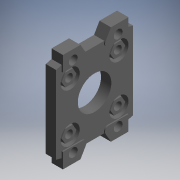
# Autodesk Inventor part: CA1-F06(F)
Saved by Autodesk Inventor 2017.3 (Build 213256000, 256)
## iProperties
Part Number: CA1-F06(F)
Material: Generic
Catalog Web Link: www.cadenas.de
Description: CE2 FLANGE-Stroke Reading Cylinder with Brake
Vendor: SMC
Document SubType Name: Modeling
Designer: partserver
Manufacturer: SMC
Mass: 122.984 g
Surface Area: 369.351 cm^2
Volume: 122.984 cm^3
Density: 1 g/cm^3
Appearance: PSOLRGB-128-128-128
Category: PARTsolutions
Company: SMC
Title: CA1-F06
Author: Cadenas PARTsolutions
Comments: Stroke Reading Cylinder with Brake
PSOL_IDENT_0: {$CADENAS_DATA\23d-libs\smc_jp\actuator\stroke_reading_cylinders\ce2\parts\ce2_flange.prj},166 {VTYP=
PSOL_IDENT_1: 3D},{NB=CA1-F06(F)},{LINA=CA1-F06},{NN=CE2 FLANGE},{DATE=05.07.2021 01:49:17},{GEOMDATE=15.05.2019 0
PSOL_IDENT_2: 8:14:22},{VERSION=},{LINEID=80},{WBVAR=MOUNT},{WBNUMERIC=}  {NB=CA1-F06(F)},{LINA=CA1-F06},{KT=DUMMY
PSOL_IDENT_3: },{PARTNO=CA1-F06},{BORE=63},{MOUNT=F},{B=85},{C=64},{D=20},{E=40},{J=M10x1.25},{JN=10},{FB=101},{FV=
PSOL_IDENT_4: 86},{FD=11.5},{FT=15},{FX=105},{FY=59},{FZ=130},{NM=6.0},{NS=17},{WM=2.0},{WD=8.70},{FT2=13.5},{FT3=
PSOL_IDENT_5: 4},{FB2=40},{FR=5},{FX2=90.2},{FZ2=102.0},{FA=75},{D0=44.000}
NB: CA1-F06(F)
NN: CE2 FLANGE
NT: Stroke Reading Cylinder with Brake
NBSYN: $PARTNO.($MOUNT.)
LINA: CA1-F06
CATALOG: SMC (JP
PARTNO: CA1-F06
BORE: 63
MOUNT: (F) Rod side flange style
B: 85
C: 64
D: 20
E: 40
J: M10x1.25
JN: 10
FB: 101
FV: 86
FD: 11.5
FT: 15
FX: 105
FY: 59
FZ: 130
NM: 6
NS: 17
WM: 2
WD: 8.7
FT2: 13.5
FT3: 4
FB2: 40
FR: 5
FX2: 90.2
FZ2: 102
FA: 75
D0: 44
SUPPLIER: SMC
ARTICLENO: CA1-F06(F)
BOMINFO: CA1-F06
CREATOR: CADENAS GmbH
Autodesk Inventor part; units mm, degrees
sketch "Sketch_1" plane through (0, 0, 0) normal (1, 0, 0) x (0, 1, 0)
  line L0 (43, 53.0096) -> (43, 52.5)
  line L1 (43, 52.5) -> (-43, 52.5)
  line L2 (-43, 52.5) -> (-43, 53.0096)
  line L3 (-43, 53.0096) -> (-50.5, 51)
  line L4 (-50.5, 51) -> (-50.5, -51)
  line L5 (-50.5, -51) -> (-43, -53.0096)
  line L6 (-43, -53.0096) -> (-43, -52.5)
  line L7 (-43, -52.5) -> (43, -52.5)
  line L8 (43, -52.5) -> (43, -53.0096)
  line L9 (43, -53.0096) -> (50.5, -51)
  line L10 (50.5, -51) -> (50.5, 51)
  line L11 (50.5, 51) -> (43, 53.0096)
  circle A0 centre (0, 0) radius 22
  constraints: 24 end point, 1 centre point
extrude "Extrusion1" add sketch "Sketch_1" against normal blind 13.5
sketch "Sketch_2" plane through (0, 0, 0) normal (1, 0, 0) x (0, 1, 0)
  line L0 (-17.171, -45.1) -> (-43, -45.1)
  line L1 (-43, -45.1) -> (-43, -65)
  line L2 (-43, -65) -> (-20, -65)
  line L3 (-20, -65) -> (-12.8409, -52.6)
  arc A0 (-12.8409, -52.6) -> (-17.171, -45.1) centre (-17.171, -50.1) ccw
  constraints: 8 end point, 2 point on circle, 1 centre point
extrude "Extrusion2" add sketch "Sketch_2" against normal blind 15
sketch "Sketch_3" plane through (0, 0, 0) normal (1, 0, 0) x (0, 1, 0)
  arc A0 (17.171, -45.1) -> (12.8409, -52.6) centre (17.171, -50.1) ccw
  line L0 (12.8409, -52.6) -> (20, -65)
  line L1 (20, -65) -> (43, -65)
  line L2 (43, -65) -> (43, -45.1)
  line L3 (43, -45.1) -> (17.171, -45.1)
  constraints: 8 end point, 2 point on circle, 1 centre point
extrude "Extrusion3" add sketch "Sketch_3" against normal blind 15
sketch "Sketch_4" plane through (0, 0, 0) normal (1, 0, 0) x (0, 1, 0)
  line L0 (-20, 65) -> (-43, 65)
  line L1 (-43, 65) -> (-43, 45.1)
  line L2 (-43, 45.1) -> (-17.171, 45.1)
  arc A0 (-17.171, 45.1) -> (-12.8409, 52.6) centre (-17.171, 50.1) ccw
  line L3 (-12.8409, 52.6) -> (-20, 65)
  constraints: 8 end point, 2 point on circle, 1 centre point
extrude "Extrusion4" add sketch "Sketch_4" against normal blind 15
sketch "Sketch_5" plane through (0, 0, 0) normal (1, 0, 0) x (0, 1, 0)
  line L0 (20, 65) -> (12.8409, 52.6)
  arc A0 (12.8409, 52.6) -> (17.171, 45.1) centre (17.171, 50.1) ccw
  line L1 (17.171, 45.1) -> (43, 45.1)
  line L2 (43, 45.1) -> (43, 65)
  line L3 (43, 65) -> (20, 65)
  constraints: 8 end point, 2 point on circle, 1 centre point
extrude "Extrusion5" add sketch "Sketch_5" against normal blind 15
sketch "Sketch6" plane through (0, 0, 0) normal (1, 0, 0) x (0, 0, -1)
  point P0 (52.5, 29.5)
hole "Hole1" at (0, 29.5, -52.5) direction (-1, 0, 0) diameter 11.5 depth 15
pattern_linear "Rectangular Pattern1" count 2 spacing 105 along (0, 0, 1) count 2 spacing 59 along (0, -1, 0) of "Hole1"
sketch "Sketch_8" plane through (0, 0, -32) normal (0, 0, 1) x (1, 0, 0)
  line L0 (-15, 32) -> (0, 32)
  line L1 (0, 32) -> (0, 27)
  line L2 (0, 27) -> (-6, 27)
  line L3 (-6, 27) -> (-6, 23.3)
  line L4 (-6, 23.3) -> (-4, 23.3)
  line L5 (-4, 23.3) -> (-4, 19.5)
  line L6 (-4, 19.5) -> (-15, 19.5)
  line L7 (-15, 19.5) -> (-15, 32)
  line L8 (-15, 32) -> (0, 32)
  constraints: 18 end point
revolve "Revolution1" cut sketch "Sketch_8" angle 360 about axis through (-15, 32, -32) along (-1, 0, 0)
pattern_linear "Rectangular Pattern2" count 2 spacing 64 along (0, 0, 1) count 2 spacing 64 along (0, -1, 0) of "Revolution1"
sketch "Sketch_10" plane through (-6, 0, 0) normal (1, 0, 0) x (0, 0, -1)
  line L0 (23.5, 27.0925) -> (32, 22.185)
  line L1 (32, 22.185) -> (40.5, 27.0925)
  line L2 (40.5, 27.0925) -> (40.5, 36.9075)
  line L3 (40.5, 36.9075) -> (32, 41.815)
  line L4 (32, 41.815) -> (23.5, 36.9075)
  line L5 (23.5, 36.9075) -> (23.5, 27.0925)
  circle A0 centre (32, 32) radius 5
  constraints: 12 end point, 1 centre point
extrude "Extrusion6" add sketch "Sketch_10" against normal blind 6
sketch "Sketch_11" plane through (-6, 0, 0) normal (1, 0, 0) x (0, 0, -1)
  line L0 (-40.5, 27.0925) -> (-32, 22.185)
  line L1 (-32, 22.185) -> (-23.5, 27.0925)
  line L2 (-23.5, 27.0925) -> (-23.5, 36.9075)
  line L3 (-23.5, 36.9075) -> (-32, 41.815)
  line L4 (-32, 41.815) -> (-40.5, 36.9075)
  line L5 (-40.5, 36.9075) -> (-40.5, 27.0925)
  circle A0 centre (-32, 32) radius 5
  constraints: 12 end point, 1 centre point
extrude "Extrusion7" add sketch "Sketch_11" against normal blind 6
sketch "Sketch_13" plane through (-6, 0, 0) normal (1, 0, 0) x (0, 0, -1)
  line L0 (-40.5, -36.9075) -> (-32, -41.815)
  line L1 (-32, -41.815) -> (-23.5, -36.9075)
  line L2 (-23.5, -36.9075) -> (-23.5, -27.0925)
  line L3 (-23.5, -27.0925) -> (-32, -22.185)
  line L4 (-32, -22.185) -> (-40.5, -27.0925)
  line L5 (-40.5, -27.0925) -> (-40.5, -36.9075)
  circle A0 centre (-32, -32) radius 5
  constraints: 12 end point, 1 centre point
extrude "Extrusion8" add sketch "Sketch_13" against normal blind 6
sketch "Sketch_14" plane through (-6, 0, 0) normal (1, 0, 0) x (0, 0, -1)
  line L0 (23.5, -36.9075) -> (32, -41.815)
  line L1 (32, -41.815) -> (40.5, -36.9075)
  line L2 (40.5, -36.9075) -> (40.5, -27.0925)
  line L3 (40.5, -27.0925) -> (32, -22.185)
  line L4 (32, -22.185) -> (23.5, -27.0925)
  line L5 (23.5, -27.0925) -> (23.5, -36.9075)
  circle A0 centre (32, -32) radius 5
  constraints: 12 end point, 1 centre point
extrude "Extrusion9" add sketch "Sketch_14" against normal blind 6
ref_plane "f_XY" through (0, 0, 0) normal (1, 0, 0) x (0, 0, -1)
ref_plane "f_YZ" through (0, 0, 0) normal (0, 0, -1) x (0, 1, 0)
ref_plane "f_ZX" through (0, 0, 0) normal (0, 1, 0) x (1, 0, 0)
body "Solid1"
